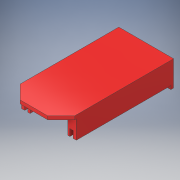
# Autodesk Inventor part: top-slider
Saved by Autodesk Inventor 2018 (Build 220112000, 112)
## iProperties
Created: 2019-10-14
Part Number: top-slider
Material: Generic
Document SubType Name: Modeling
Designer: jklei
Density: 1 g/cm^3
Appearance: Default
Author: jklei
Autodesk Inventor part; units mm, degrees
ref_plane "YZ Plane" through (0, 0, 0) normal (1, 0, 0) x (0, 1, 0)
ref_plane "XZ Plane" through (0, 0, 0) normal (0, 1, 0) x (-1, 0, 0)
ref_plane "XY Plane" through (0, 0, 0) normal (0, 0, 1) x (1, 0, 0)
sketch "Sketch1" plane through (0, 0, 0) normal (0, 0, 1) x (1, 0, 0)
  line L0 (0, 0) -> (0, 6.35)
  line L1 (0, 6.35) -> (-3.048, 6.35)
  line L2 (1.905, 0) -> (1.905, 12.7)
  line L3 (-3.048, 0) -> (-5.969, 0)
  line L4 (-5.969, 0) -> (-5.969, 15.875)
  line L5 (44.831, 0) -> (41.91, 0)
  line L6 (41.91, 6.35) -> (38.862, 6.35)
  line L7 (38.862, 6.35) -> (38.862, 0)
  line L8 (38.862, 0) -> (36.957, 0)
  line L9 (36.957, 0) -> (36.957, 12.7)
  line L10 (0, 0) -> (1.905, 0)
  line L11 (44.831, 0) -> (44.831, 15.875)
  line L12 (-3.048, 6.35) -> (-3.048, 0)
  line L13 (41.91, 6.35) -> (41.91, 0)
  line L14 (44.831, 15.875) -> (44.831, 20.32)
  line L15 (44.831, 20.32) -> (-5.969, 20.32)
  line L16 (-5.969, 20.32) -> (-5.969, 15.875)
  line L17 (1.905, 12.7) -> (1.905, 17.145)
  line L18 (1.905, 17.145) -> (36.957, 17.145)
  line L19 (36.957, 17.145) -> (36.957, 12.7)
  dimension "d3" = 6.35
  dimension "d4" = 3.048
  dimension "d9" = 1.905
  dimension "d10" = 12.7
  dimension "d15" = 50.8
  dimension "d18" = 15.875
  dimension "d19" = 15.875
  dimension "d21" = 6.35
  dimension "d22" = 3.048
  dimension "d23" = 1.905
  dimension "d24" = 12.7
  dimension "d25" = 35.052
  dimension "d26" = 2.921
  dimension "d27" = 2.921
  dimension "d39" = 4.445
  dimension "d40" = 4.445
  constraints: 40 end point, 7 perpendicular, 6 vertical, 4 horizontal, 1 collinear
  measures "d3" distance of L0.start L0.end
  measures "d4" distance of L0.end L1.end
  measures "d9" distance of L0.start L2.start
  measures "d10" distance of L2.start L2.end
  measures "d15" distance of L11.end L4.end
  measures "d18" distance of L11.end L5.start
  measures "d19" distance of L3.end L4.end
  measures "d21" distance of L5.end L6.start
  measures "d22" distance of L6.start L6.end
  measures "d23" distance of L7.end L8.end
  measures "d24" distance of L8.end L9.end
  measures "d25" distance of L2.end L9.end
  measures "d26" distance of L3.start L3.end
  measures "d27" distance of L5.start L5.end
  measures "d39" distance of L11.end L14.end
  measures "d40" distance of L2.end L17.end
extrude "Extrusion1" add sketch "Sketch1" along normal blind 91.44
sketch "Sketch2" plane through (0, 0, 91.44) normal (0, 0, 1) x (1, 0, 0)
  line L0 (1.905, 17.145) -> (-5.9455, 17.145)
  line L1 (36.957, 17.145) -> (1.905, 17.145) projected
  line L2 (36.957, 17.145) -> (44.831, 17.145)
  line L3 (44.831, 20.32) -> (44.831, 0) projected
  line L4 (44.831, 20.32) -> (-5.969, 20.32) projected
  line L5 (-5.969, 20.32) -> (44.831, 20.32)
  line L6 (44.831, 20.32) -> (44.831, 17.145)
  line L7 (44.831, 17.145) -> (-5.969, 17.145)
  line L8 (-5.969, 17.145) -> (-5.969, 20.32)
  point P0 (0, 0)
  constraints: 12 end point, 3 horizontal, 2 parallel, 1 perpendicular, 1 point on line
extrude "Extrusion2" add sketch "Sketch2" along normal blind 14.0208
chamfer "Chamfer1" distance 12.7 angle 45 2 edges at (44.831, 18.7325, 105.4608) (-5.969, 18.7325, 105.4608)
sketch "Sketch3" plane through (0, 0, 0) normal (0, 0, -1) x (-1, 0, 0)
  line L0 (0, 0) -> (0, 6.35) projected
  line L1 (0, 6.35) -> (3.048, 6.35) projected
  line L2 (3.048, 6.35) -> (3.048, 0) projected
  line L3 (3.048, 0) -> (5.969, 0) projected
  line L4 (5.969, 0) -> (5.969, 20.32) projected
  line L5 (-44.831, 20.32) -> (-44.831, 0) projected
  line L6 (-44.831, 0) -> (-41.91, 0) projected
  line L7 (-41.91, 0) -> (-41.91, 6.35) projected
  line L8 (-41.91, 6.35) -> (-38.862, 6.35) projected
  line L9 (-38.862, 6.35) -> (-38.862, 0) projected
  line L10 (-38.862, 0) -> (-36.957, 0) projected
  line L11 (-36.957, 0) -> (-36.957, 17.145) projected
  line L12 (-1.905, 17.145) -> (-1.905, 0) projected
  line L13 (-1.905, 0) -> (0, 0) projected
  line L14 (5.969, 20.32) -> (-44.831, 20.32) projected
  line L15 (-36.957, 17.145) -> (-1.905, 17.145) projected
extrude "Extrusion3" cut sketch "Sketch3" against normal blind 3.81
sketch "Sketch4" plane through (0, 0, 3.81) normal (0, 0, -1) x (-1, 0, 0)
  line L0 (5.969, 15.875) -> (5.969, 0)
  line L1 (-44.831, -3.175) -> (5.969, -3.175)
  line L2 (5.969, -3.175) -> (5.969, 0)
  line L3 (-44.831, 20.32) -> (-32.131, 20.32) projected
  line L4 (-44.831, -3.175) -> (-44.831, 20.32)
  line L5 (-6.731, 20.32) -> (5.969, 20.32) projected
  line L6 (-44.831, 20.32) -> (5.969, 20.32)
  line L7 (5.969, 20.32) -> (5.969, 15.875)
  point P0 (0, 0)
  constraints: 12 end point, 3 perpendicular, 1 vertical
extrude "Extrusion4" add sketch "Sketch4" along normal blind 2.54
body "Solid1"
